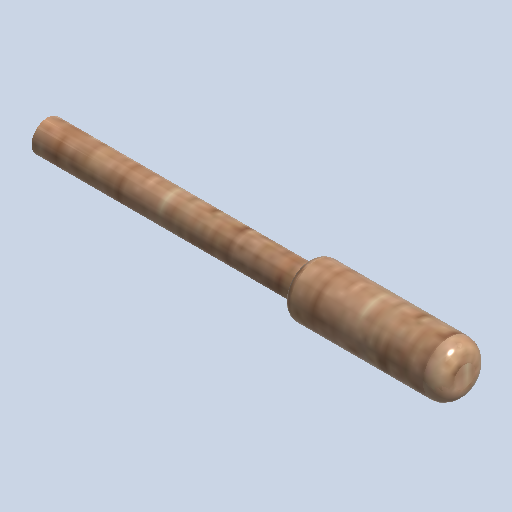
# Autodesk Inventor part: ocas
Saved by Autodesk Inventor 2025.2 (Build 292293000, 293)
## iProperties
Part Number: ocas
Material: Wood (Birch)
Document SubType Name: Modeling
Designer: fanda
Appearance: Birch - Natural Polished
Density: 0.55 g/cm^3
Author: fanda
Autodesk Inventor part; units mm, degrees
ref_plane "YZ Plane" through (0, 0, 0) normal (1, 0, 0) x (0, 1, 0)
ref_plane "XZ Plane" through (0, 0, 0) normal (0, 1, 0) x (-1, 0, 0)
ref_plane "XY Plane" through (0, 0, 0) normal (0, 0, 1) x (1, 0, 0)
sketch "Sketch1" plane through (0, 0, 0) normal (0, 0, 1) x (1, 0, 0)
  line L0 (-10.014, 0) -> (-10.014, 3)
  line L1 (-10.014, 3) -> (39.986, 3)
  line L2 (39.986, 3) -> (39.986, 3.5)
  line L3 (41.486, 5) -> (66.986, 5)
  line L4 (69.986, 2) -> (69.986, 0)
  arc A0 (41.486, 5) -> (39.986, 3.5) centre (41.486, 3.5) ccw
  arc A1 (69.986, 2) -> (66.986, 5) centre (66.986, 2) ccw
  line L5 (-10.014, 0) -> (69.986, 0)
  point P0 (0, 0)
  point P1 (39.986, 5)
  point P2 (69.986, 5)
  dimension "d0" = 3
  dimension "d1" = 50
  dimension "d2" = 2
  dimension "d3" = 30
  dimension "d4" = 1.5
  dimension "d5" = 3
  constraints: 12 end point, 4 perpendicular, 4 point on circle, 4 point on line, 4 tangent, 2 centre point, 1 horizontal, 1 vertical
  measures "d0" distance of L0.start L0.end
  measures "d1" distance of L0.end L1.end
  measures "d2" distance of L1.end point (39.986, 5)
  measures "d3" distance of point (39.986, 5) point (69.986, 5)
  measures "d4" radius of A0
  measures "d5" radius of A1
revolve "Revolution1" add sketch "Sketch1" angle 360 about axis through (-10.014, 0, 0) along (1, 0, 0)
